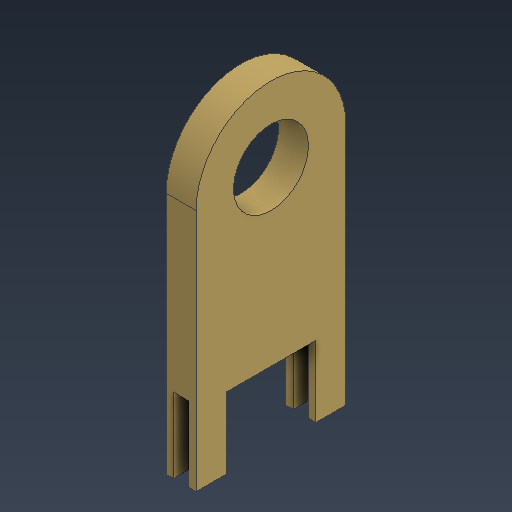
# Autodesk Inventor part: Terminais
Saved by Autodesk Inventor 2021 (Build 250183000, 183)
## iProperties
Created: 2021-01-23
Part Number: Terminais
Material: Genérico
Document SubType Name: Modeling
Designer: João
Density: 1 g/cm^3
Appearance: Padrão
Author: João
Autodesk Inventor part; units mm, degrees
ref_plane "YZ Plane" through (0, 0, 0) normal (1, 0, 0) x (0, 1, 0)
ref_plane "XZ Plane" through (0, 0, 0) normal (0, 1, 0) x (-1, 0, 0)
ref_plane "XY Plane" through (0, 0, 0) normal (0, 0, 1) x (1, 0, 0)
sketch "Esboço1" plane through (0, 0, 0) normal (0, 1, 0) x (-1, 0, 0)
  line L0 (0.2, 1) -> (-0.2, 1)
  line L1 (-0.2, 1) -> (-0.2, -1)
  line L2 (-0.2, -1) -> (0.2, -1)
  line L3 (0.2, -1) -> (0.2, 1)
  line L4 (0.2, 1) -> (-0.2, -1) construction
  line L5 (-0.2, 1) -> (0.2, -1) construction
  point P0 (0, 0)
  dimension "d0" = 0.4
  dimension "d1" = 2
  constraints: 12 end point, 2 midpoint, 2 parallel, 1 horizontal, 1 perpendicular
  measures "d0" distance of L2.end L1.end
  measures "d1" distance of L1.end L0.end
extrude "Extrusão1" add sketch "Esboço1" along normal blind 4.25
sketch "Esboço2" plane through (0.2, 0, 1) normal (1, 0, 0) x (0, 0, -1)
  line L0 (0, 4.25) -> (2, 4.25) projected
  line L1 (1, 4.25) -> (1, 3.25)
  circle A0 centre (1, 3.25) radius 0.5
  point P0 (1, 0)
  dimension "d4" = 1
  dimension "d5" = 1
  constraints: 2 end point, 1 centre point, 1 coincident, 1 midpoint, 1 vertical
  measures "d4" distance of L1.start L1.end
  measures "d5" diameter of A0
extrude "Extrusão2" cut sketch "Esboço2" against normal blind 4.25
fillet "Arredondamento1" radius 1 2 edges at (0, 4.25, 1) (0, 4.25, -1)
sketch "Esboço3" plane through (0, 0, 0) normal (0, -1, 0) x (1, 0, 0)
  line L0 (0.2, 1) -> (0.2, -1) projected
  line L1 (-0.2, 0.6) -> (0.2, 0.6)
  line L2 (0.2, 0.6) -> (0.2, -0.6)
  line L3 (0.2, -0.6) -> (-0.2, -0.6)
  line L4 (-0.2, -0.6) -> (-0.2, 0.6)
  line L5 (-0.2, 0.6) -> (0.2, -0.6) construction
  line L6 (0.2, 0.6) -> (-0.2, -0.6) construction
  point P0 (0, 0)
  dimension "d9" = 1.2
  constraints: 12 end point, 2 midpoint, 2 parallel, 1 horizontal, 1 perpendicular, 1 point on line
  measures "d9" distance of L1.end L2.end
extrude "Extrusão3" cut sketch "Esboço3" against normal blind 0.95
sketch "Esboço4" plane through (0, 0, 0) normal (0, -1, 0) x (1, 0, 0)
  line L0 (0.2, -0.6) -> (-0.2, -0.6) projected
  line L1 (0.1, -1) -> (-0.1, -1)
  line L2 (-0.1, -1) -> (-0.1, -0.6)
  line L3 (-0.1, -0.6) -> (0.1, -0.6)
  line L4 (0.1, -0.6) -> (0.1, -1)
  line L5 (0.1, -1) -> (-0.1, -0.6) construction
  line L6 (-0.1, -1) -> (0.1, -0.6) construction
  line L7 (-0.2, -0.5) -> (-0.2, 0.5) projected
  line L8 (-0.2, 0) -> (0.2, 0)
  line L9 (0.2, 0.5) -> (0.2, -0.5) projected
  line L10 (0.2, 0.6) -> (-0.2, 0.6)
  line L11 (0.1, 1) -> (-0.1, 1)
  line L12 (-0.1, 1) -> (-0.1, 0.6)
  line L13 (-0.1, 0.6) -> (0.1, 0.6)
  line L14 (0.1, 0.6) -> (0.1, 1)
  line L15 (0.1, 1) -> (-0.1, 0.6) construction
  line L16 (-0.1, 1) -> (0.1, 0.6) construction
  line L17 (-0.2, -1) -> (-0.2, -0.6) projected
  point P0 (0, 0)
  point P1 (0, -0.8)
  point P2 (0, 0.8)
  point P3 (0.1, -0.6)
  point P4 (0.1, 0.6)
  dimension "d12" = 0.2
  dimension "d15" = 0.1
  constraints: 28 end point, 7 symmetric about line, 6 midpoint, 2 horizontal, 2 parallel, 2 point on line, 1 perpendicular
  measures "d12" distance of L2.end L3.end
  measures "d15" distance between parallel lines of L17 L2
extrude "Extrusão4" cut sketch "Esboço4" against normal blind 1
